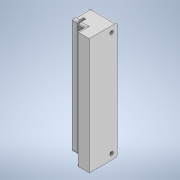
# Autodesk Inventor part: Wal Mount
Saved by Autodesk Inventor 2020.2 (Build 242310000, 310)
## iProperties
Created: 2019-12-20
Part Number: Wal Mount
Material: Generic
Document SubType Name: Modeling
Designer: Cosmin Rotaru
Density: 1 g/cm^3
Appearance: Default
Author: Cosmin Rotaru
Autodesk Inventor part; units mm, degrees
ref_plane "YZ Plane" through (0, 0, 0) normal (1, 0, 0) x (0, 1, 0)
ref_plane "XZ Plane" through (0, 0, 0) normal (0, 1, 0) x (-1, 0, 0)
ref_plane "XY Plane" through (0, 0, 0) normal (0, 0, 1) x (1, 0, 0)
sketch "Sketch1" plane through (0, 0, 0) normal (0, 1, 0) x (-1, 0, 0)
  line L0 (47.4221, 0) -> (47.4221, -5)
  line L1 (47.4221, -5) -> (45.5221, -5)
  line L2 (45.5221, -5) -> (45.5221, 1)
  line L3 (47.4221, 0) -> (52.4221, 0)
  line L4 (52.4221, 0) -> (52.4221, -12)
  line L5 (52.4221, -12) -> (29.5221, -12)
  line L6 (45.5221, 1) -> (40.5221, 1)
  line L7 (29.5221, -12) -> (29.5221, 8)
  line L8 (29.5221, 8) -> (40.5221, 8)
  line L9 (40.5221, 8) -> (40.5221, 1)
  line L10 (47.4221, -5) -> (52.4221, -5)
  line L11 (52.4221, -5) -> (52.4221, -16)
  line L12 (52.4221, -16) -> (29.5221, -16)
  line L13 (29.5221, -16) -> (29.5221, -12)
  point P0 (0, 0)
  dimension "d0" = 5
  dimension "d1" = 1.9
  dimension "d2" = 6
  dimension "d4" = 5
  dimension "d5" = 12
  dimension "d6" = 5
  dimension "d7" = 20
  dimension "d8" = 11
  dimension "d9" = 7
  dimension "d10" = 11
  constraints: 28 end point, 9 perpendicular, 2 point on line, 2 vertical, 1 horizontal
  measures "d0" distance of L0.start L0.end
  measures "d1" distance of L0.end L1.end
  measures "d2" distance of L1.end L2.end
  measures "d4" distance of L0.start L3.end
  measures "d5" distance of L3.end L4.end
  measures "d6" distance of L2.end L6.end
  measures "d7" distance of L5.end L7.end
  measures "d8" distance of L7.end L8.end
  measures "d9" distance of L8.end L6.end
  measures "d10" distance of L10.end L11.end
extrude "Extrusion1" add sketch "Sketch1" along normal blind 100
sketch "Sketch2" plane through (-52.4221, 0, -16) normal (-1, 0, 0) x (0, 0, 1)
  line L0 (0, 0) -> (0, 100) projected
  line L1 (0, 0) -> (5, 0)
  line L2 (24, 0) -> (0, 0) projected
  line L3 (5, 0) -> (5, 5)
  circle A0 centre (5, 5) radius 1.5
  line L4 (0, 100) -> (5, 100)
  line L5 (24, 100) -> (0, 100) projected
  line L6 (5, 100) -> (5, 95)
  circle A1 centre (5, 95) radius 1.5
  point P0 (16, 0)
  dimension "d13" = 5
  dimension "d14" = 5
  dimension "d15" = 3
  dimension "d16" = 5
  dimension "d17" = 5
  dimension "d18" = 3
  constraints: 8 end point, 2 centre point, 2 coincident, 2 perpendicular, 2 point on line
  measures "d13" distance of L0.start L1.end
  measures "d14" distance of L1.end L3.end
  measures "d15" diameter of A0
  measures "d16" distance of L0.end L4.end
  measures "d17" distance of L4.end L6.end
  measures "d18" diameter of A1
hole "Hole1" at (-52.4221, 5, -11) at (-52.4221, 95, -11) direction (1, 0, 0) diameter 3 end through all
fillet "Fillet1" radius 2 12 edges at (-52.4221, 50, -16) (-52.4221, 0, -8) (-52.4221, 100, -8) (-40.9721, 100, -16) (-40.9721, 0, -16) (-40.5221, 50, 8) (-40.5221, 0, 4.5) (-43.0221, 0, 1) (-49.9221, 0, 0) (-49.9221, 100, 0) (-43.0221, 100, 1) (-40.5221, 100, 4.5)
body "Solid1"
